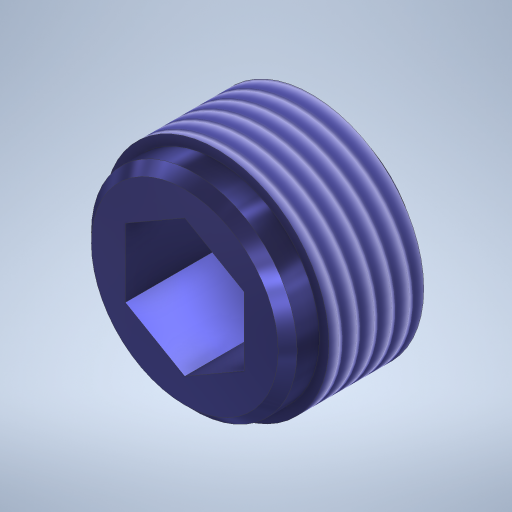
# Autodesk Inventor part: Pillow Ball Retainer
Saved by Autodesk Inventor 2023.1 (Build 271208000, 208)
## iProperties
Created: 2019-11-25
Part Number: Pillow Ball Retainer
Material: Generic
Document SubType Name: Modeling
Designer: Jopa
Density: 1 g/cm^3
Appearance: Poplar
Author: Jopa
Autodesk Inventor part; units mm, degrees
ref_plane "YZ Plane" through (0, 0, 0) normal (1, 0, 0) x (0, 1, 0)
ref_plane "XZ Plane" through (0, 0, 0) normal (0, 1, 0) x (-1, 0, 0)
ref_plane "XY Plane" through (0, 0, 0) normal (0, 0, 1) x (1, 0, 0)
sketch "Sketch1" plane through (0, 0, 0) normal (0, 0, 1) x (1, 0, 0)
  circle A0 centre (0, 0) radius 4.5085
  dimension "d0" = 9.017
  constraints: 1 centre point, 1 coincident
  measures "d0" diameter of A0
extrude "Extrusion1" add sketch "Sketch1" along normal blind 5.08
sketch "Sketch2" plane through (0, 0, 0) normal (0, 0, -1) x (-1, 0, 0)
  circle A0 centre (0, 0) radius 3.81
  dimension "d3" = 7.62
  constraints: 1 centre point, 1 coincident
  measures "d3" diameter of A0
extrude "Extrusion2" add sketch "Sketch2" along normal blind 0.635 draft -15
sketch "Sketch3" plane through (0, 0, 5.08) normal (0, 0, 1) x (1, 0, 0)
  circle A0 centre (0, 0) radius 4.1275
  circle A1 centre (0, 0) radius 4.5085 projected
  dimension "d6" = 8.255
  constraints: 1 centre point, 1 coincident
  measures "d6" diameter of A0
extrude "Extrusion3" cut sketch "Sketch3" against normal blind 1.27
chamfer "Chamfer1" distance 0.381 angle 45 1 edges at (-4.1275, 0, 5.08)
sketch "Sketch4" plane through (0, 0, 5.08) normal (0, 0, 1) x (1, 0, 0)
  circle A0 centre (0, 0) radius 2.3813 construction
  line L0 (-2.3813, 1.3748) -> (0, 2.7496)
  line L1 (0, 2.7496) -> (2.3812, 1.3748)
  line L2 (2.3812, 1.3748) -> (2.3813, -1.3748)
  line L3 (2.3813, -1.3748) -> (0, -2.7496)
  line L4 (0, -2.7496) -> (-2.3812, -1.3748)
  line L5 (-2.3812, -1.3748) -> (-2.3813, 1.3748)
  point P0 (-2.3813, 0)
  dimension "d12" = 4.7625
  constraints: 12 end point, 2 coincident, 1 horizontal alignment, 1 midpoint, 1 vertical, 15 other
extrude "Extrusion4" cut sketch "Sketch4" against normal through all
thread "Thread1" size "3/8-36 UNS" class "2A" standard "ANSI Unified Screw Threads" full length
body "Solid1"
